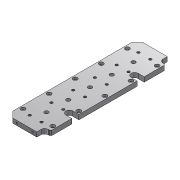
# Autodesk Inventor part: BC-10017
Saved by Autodesk Inventor 2016 (Build 200138000, 138)
## iProperties
Created: 2015-11-11
Part Number: BC-10017
Project: DIPOLO BC-3T- SIRIUS
Cost Center: 1504002005
Material: Alumínio 7075
Document SubType Name: Modeling
Designer: reinaldo.basilio
Density: 2.81 g/cm^3
Appearance: Aluminum - Polished
Mass: 879.544 g
Surface Area: 742.713 cm^2
Volume: 313.005 cm^3
Description: Suporte de fixação entre a base e o polo de baixo campo.
RuleStatus: InUse
AfterMaterialChange0: file://_iMaterial
AfterAnyiPropertyChange0: file://_iMaterial
AfterDocNew0: file://_Naming_par
AfterDocNew1: file://_NameStart
AfterDocNew2: file://_NameStart1
AfterDocNew3: file://_Materiais
DocNumber: XXXXX-XXX-XXXX-00-001.ipt
Folder: .
Title: DIPOLO BC-3T- SIRIUS
Author: reinaldo.basilio
Subject: BC-10017
Autodesk Inventor part; units mm, degrees
ref_plane "YZ Plane" through (0, 0, 0) normal (1, 0, 0) x (0, 1, 0)
ref_plane "XZ Plane" through (0, 0, 0) normal (0, 1, 0) x (-1, 0, 0)
ref_plane "XY Plane" through (0, 0, 0) normal (0, 0, 1) x (1, 0, 0)
sketch "Sketch5" plane through (0, 0, 0) normal (0, 0, 1) x (1, 0, 0)
  line L0 (-165, 45.5) -> (165, 45.5)
  line L1 (165, 45.5) -> (165, -45.5)
  line L2 (165, -45.5) -> (-165, -45.5)
  line L3 (-165, -45.5) -> (-165, 45.5)
  point P0 (0, 0)
  point P1 (0, 45.5)
  point P2 (165, 0)
  dimension "d8" = 330
  dimension "d9" = 91
  constraints: 8 end point, 2 midpoint, 2 parallel, 1 horizontal, 1 horizontal alignment, 1 perpendicular, 1 vertical alignment
  measures "d8" distance of L0.start L0.end
  measures "d9" distance of L2.end L0.start
extrude "Extrusion5" add sketch "Sketch5" along normal mid plane 12
sketch "Sketch6" plane through (0, 0, 6) normal (0, 0, 1) x (1, 0, 0)
  circle A0 centre (132, -37.5) radius 3
  circle A1 centre (66, -37.5) radius 3
  circle A2 centre (-66, -37.5) radius 3
  circle A3 centre (-132, -37.5) radius 3
  circle A4 centre (0, -37.5) radius 3
  circle A5 centre (132, 37.75) radius 3
  circle A6 centre (66, 37.75) radius 3
  circle A7 centre (-66, 37.75) radius 3
  circle A8 centre (-132, 37.75) radius 3
  circle A9 centre (0, 37.75) radius 3
  line L0 (165, 45.5) -> (-165, 45.5) projected
  circle A10 centre (132, -37.5) radius 5
  point P0 (-165, -45.5)
  point P1 (0, 0)
  dimension "d12" = 66
  dimension "d13" = 66
  dimension "d14" = 66
  dimension "d17" = 6
  dimension "d20" = 66
  dimension "d22" = 66
  dimension "d23" = 66
  dimension "d24" = 66
  dimension "d25" = 6
  dimension "d26" = 66
  dimension "d27" = 75.25
  dimension "d64" = 7.75
  dimension "d65" = 91
  dimension "d103" = 10
  constraints: 11 centre point, 8 equal radius, 8 horizontal alignment, 3 coincident, 2 vertical alignment
  measures "d12" distance of point (0, -37.5) A2.centre
  measures "d13" distance of A0.centre A1.centre
  measures "d14" distance of A3.centre A2.centre
  measures "d17" diameter of A0
  measures "d20" distance of A4.centre A1.centre
  measures "d22" distance of point (0, 37.75) A7.centre
  measures "d23" distance of A5.centre A6.centre
  measures "d24" distance of A8.centre A7.centre
  measures "d25" diameter of A5
  measures "d26" distance of A9.centre A6.centre
  measures "d27" distance of A8.centre A3.centre
  measures "d64" distance from line of L0 A8.centre
  measures "d65" distance of L0.end point (-165, -45.5)
  measures "d103" diameter of A10
hole "Hole1" at (-132, 37.75, 6) at (132, 37.75, 6) at (66, 37.75, 6) at (0, 37.75, 6) at (-66, 37.75, 6) at (132, -37.5, 6) at (66, -37.5, 6) at (0, -37.5, 6) at (-66, -37.5, 6) at (-132, -37.5, 6) direction (0, 0, -1) diameter 7 end through all counterbore diameter 11 counterbore depth 6 clearance for "Socket Head Cap Screw DIN EN ISO 4762" size "M6" standard "DIN"
sketch "Sketch7" plane through (0, 0, 6) normal (0, 0, 1) x (1, 0, 0)
  line L0 (-165, 45.5) -> (-165, -45.5) projected
  line L1 (-165, -45.5) -> (165, -45.5) projected
  line L2 (165, -45.5) -> (165, 45.5) projected
  circle A0 centre (137.5, -15) radius 4
  circle A1 centre (137.5, 15) radius 4
  circle A2 centre (82.5, -15) radius 4
  circle A3 centre (82.5, 15) radius 4
  circle A4 centre (27.5, -15) radius 4
  circle A5 centre (27.5, 15) radius 4
  circle A6 centre (-27.5, -15) radius 4
  circle A7 centre (-27.5, 15) radius 4
  circle A8 centre (-82.5, -15) radius 4
  circle A9 centre (-82.5, 15) radius 4
  circle A10 centre (-137.5, -15) radius 4
  circle A11 centre (-137.5, 15) radius 4
  point P0 (0, 0)
  dimension "d35" = 27.5
  dimension "d36" = 30
  dimension "d37" = 15
  dimension "d38" = 8
  dimension "d41" = 55
  dimension "d46" = 27.5
  constraints: 12 centre point, 1 equal radius, 1 horizontal, 1 vertical alignment, 20 other
  measures "d35" distance from line of A0.centre L2
  measures "d36" distance of A1.centre A0.centre
  measures "d37" vertical distance of point (0, 0) A0.centre
  measures "d38" diameter of A0
  measures "d41" distance of A0.centre A2.centre
  measures "d46" distance from line of L0 A10.centre
hole "Hole2" at (137.5, -15, 6) at (137.5, 15, 6) at (82.5, 15, 6) at (82.5, -15, 6) at (27.5, -15, 6) at (27.5, 15, 6) at (-27.5, 15, 6) at (-27.5, -15, 6) at (-82.5, -15, 6) at (-82.5, 15, 6) at (-137.5, 15, 6) at (-137.5, -15, 6) direction (0, 0, -1) diameter 6.647 end through all thread size "M8x1.25" class "6H" standard "ISO Metric profile"
sketch "Sketch8" plane through (-165, -45.5, 6) normal (-1, 0, 0) x (0, 0, 1)
  line L0 (-12, 0) -> (-12, 91) projected
  line L1 (-11.5, 14.5) -> (-12, 14.5)
  line L2 (-12, 14.5) -> (-12, 76.5)
  line L3 (-12, 76.5) -> (-11.5, 76.5)
  line L4 (-11.5, 76.5) -> (-11.5, 14.5)
  point P0 (-6, 45.5)
  point P1 (-11.5, 45.5)
  dimension "d54" = 0.5
  dimension "d55" = 62
  constraints: 8 end point, 2 parallel, 1 collinear, 1 horizontal, 1 horizontal alignment, 1 midpoint, 1 perpendicular
  measures "d54" distance between parallel lines of L0 L4
  measures "d55" distance of L3.end L1.start
extrude "Extrusion6" cut sketch "Sketch8" against normal through all
sketch "Sketch9" plane through (0, 0, 6) normal (0, 0, 1) x (1, 0, 0)
  circle A0 centre (66, 37.75) radius 3.5
  line L0 (165, 45.5) -> (-165, 45.5)
  line L1 (82.5, 30.5) -> (82.5, 60.5) construction
  line L2 (91.5, 30.5) -> (91.5, 60.5)
  line L3 (73.5, 60.5) -> (73.5, 30.5)
  arc A1 (73.5, 30.5) -> (91.5, 30.5) centre (82.5, 30.5) ccw
  arc A2 (91.5, 60.5) -> (73.5, 60.5) centre (82.5, 60.5) ccw
  line L4 (0, 0) -> (0, 10.6364) construction
  line L5 (0, 0) -> (-13.5916, 0) construction
  line L6 (-82.5, 30.5) -> (-82.5, 60.5) construction
  line L7 (-91.5, 30.5) -> (-91.5, 60.5)
  line L8 (-73.5, 60.5) -> (-73.5, 30.5)
  arc A3 (-91.5, 30.5) -> (-73.5, 30.5) centre (-82.5, 30.5) ccw
  arc A4 (-73.5, 60.5) -> (-91.5, 60.5) centre (-82.5, 60.5) ccw
  circle A5 centre (-137.5, 15) radius 3.3235 projected
  circle A6 centre (-82.5, -15) radius 3.3235 projected
  circle A7 centre (-27.5, 15) radius 3.3235 projected
  circle A8 centre (27.5, -15) radius 3.3235 projected
  circle A9 centre (82.5, 15) radius 3.3235 projected
  circle A10 centre (137.5, -15) radius 3.3235 projected
  circle A11 centre (137.5, 15) radius 3.3235 projected
  circle A12 centre (82.5, -15) radius 3.3235 projected
  circle A13 centre (27.5, 15) radius 3.3235 projected
  circle A14 centre (-27.5, -15) radius 3.3235 projected
  circle A15 centre (-82.5, 15) radius 3.3235 projected
  circle A16 centre (-137.5, -15) radius 3.3235 projected
  circle A17 centre (-66, -37.5) radius 5.5 projected
  circle A18 centre (66, -37.5) radius 5.5 projected
  circle A19 centre (-66, 37.75) radius 5.5 projected
  circle A20 centre (66, 37.75) radius 5.5 projected
  circle A21 centre (-132, 37.75) radius 5.5 projected
  circle A22 centre (132, 37.75) radius 5.5 projected
  circle A23 centre (0, 37.75) radius 5.5 projected
  circle A24 centre (132, -37.5) radius 5.5 projected
  circle A25 centre (0, -37.5) radius 5.5 projected
  circle A26 centre (-132, -37.5) radius 5.5 projected
  line L9 (165, 45.5) -> (-165, 45.5) projected
  line L10 (-165, 45.5) -> (-165, -45.5) projected
  line L11 (-165, -45.5) -> (165, -45.5) projected
  line L12 (165, -45.5) -> (165, 45.5) projected
  point P0 (82.5, 45.5)
  point P1 (-82.5, 45.5)
  dimension "d58" = 16.5
  dimension "d59" = 30
  dimension "d61" = 18
  constraints: 22 end point, 8 point on circle, 7 symmetric about line, 5 centre point, 4 tangent, 2 vertical, 1 horizontal, 1 midpoint, 1 parallel, 1 point on line, 2 other
  measures "d58" horizontal distance of A0.centre point (82.5, 45.5)
  measures "d59" distance of L1.start L1.end
  measures "d61" distance between parallel lines of L3 L2
extrude "Extrusion7" cut sketch "Sketch9" against normal through all contours L2 A1 L3 L0 | L0 L3 A2 L2 | L8 A3 L7 L0 | L0 L7 A4 L8
sketch "Sketch10" plane through (0, 0, 6) normal (0, 0, 1) x (1, 0, 0)
  line L0 (-165, -45.5) -> (165, -45.5) projected
  line L1 (165, -45.5) -> (165, 45.5) projected
  circle A0 centre (110, 0) radius 5
  circle A1 centre (55, 0) radius 5
  circle A2 centre (0, 0) radius 5
  circle A3 centre (-55, 0) radius 5
  circle A4 centre (-110, 0) radius 5
  dimension "d66" = 55
  dimension "d70" = 55
  dimension "d75" = 10
  constraints: 5 centre point, 1 horizontal, 1 horizontal alignment, 8 other
  measures "d66" distance from line of L1 A0.centre
  measures "d70" distance of A0.centre A1.centre
  measures "d75" diameter of A0
hole "Hole3" at (110, 0, 6) at (55, 0, 6) at (0, 0, 6) at (-55, 0, 6) at (-110, 0, 6) direction (0, 0, -1) diameter 10 end through all
sketch "Sketch11" plane through (165, -31, -5.5) normal (1, 0, 0) x (0, 0, -1)
  circle A0 centre (-5.5, 11) radius 3
  circle A1 centre (-5.5, 51) radius 3
  point P0 (-5.5, 31)
  dimension "d86" = 40
  dimension "d87" = 20
  dimension "d88" = 6
  constraints: 2 centre point, 2 vertical alignment, 1 equal radius
  measures "d86" distance of A1.centre A0.centre
  measures "d87" distance of A1.centre point (-5.5, 31)
  measures "d88" diameter of A1
hole "Hole4" at (165, -20, 0) at (165, 20, 0) direction (-1, 0, 0) diameter 4.134 depth 15 tip angle 118 thread size "M5x0.8" class "6H" standard "ISO Metric profile"
sketch "Sketch12" plane through (-165, -31, -5.5) normal (-1, 0, 0) x (0, 0, 1)
  circle A0 centre (5.5, 11) radius 2.067
  circle A1 centre (5.5, 51) radius 2.067
  circle A2 centre (5.5, 11) radius 2.067 projected
  circle A3 centre (5.5, 51) radius 2.067 projected
  point P0 (5.5, 31)
  constraints: 4 concentric, 2 centre point, 2 vertical alignment
hole "Hole5" at (-165, -20, 0) at (-165, 20, 0) direction (1, 0, 0) diameter 4.134 depth 15 tip angle 118 thread size "M5x0.8" class "6H" standard "ISO Metric profile"
chamfer "Chamfer2" distance 15 angle 45 2 edges at (165, -45.5, 0) (-165, -45.5, 0)
sketch "Sketch13" plane through (0, 0, 6) normal (0, 0, 1) x (1, 0, 0)
  circle A0 centre (0, 37.75) radius 5.5 projected
  line L0 (165, 45.5) -> (145, 45.5)
  line L1 (145, 45.5) -> (145, 30.5)
  line L2 (145, 30.5) -> (165, 30.5)
  line L3 (165, 30.5) -> (165, 45.5)
  line L4 (0, 37.75) -> (0, 63.3817) construction
  line L5 (-165, 45.5) -> (-145, 45.5)
  line L6 (-145, 45.5) -> (-145, 30.5)
  line L7 (-145, 30.5) -> (-165, 30.5)
  line L8 (-165, 30.5) -> (-165, 45.5)
  dimension "d107" = 15
  dimension "d108" = 20
  constraints: 18 end point, 3 symmetric about line, 2 parallel, 1 horizontal, 1 perpendicular, 1 vertical
  measures "d107" distance of L0.end L1.end
  measures "d108" distance of L1.end L2.end
extrude "Extrusion8" cut sketch "Sketch13" against normal through all contours L3 L2 L1 L0 | L5 L6 L7 L8
fillet "Fillet1" radius 9 2 edges at (145, 30.5, 0.25) (-145, 30.5, 0.25)
chamfer "Chamfer3" distance 3 angle 45 2 edges at (145, 45.5, 0) (-145, 45.5, 0)
equation "\"d13\" = d12"
equation "\"d14\" = d12"
equation "\"d20\" = d12"
equation "\"d23\" = d22"
equation "\"d24\" = d22"
equation "\"d26\" = d22"
equation "\"d37\" = 0.5 * d36"
equation "\"d87\" = 0.5 * d86"
body "Solid5"
